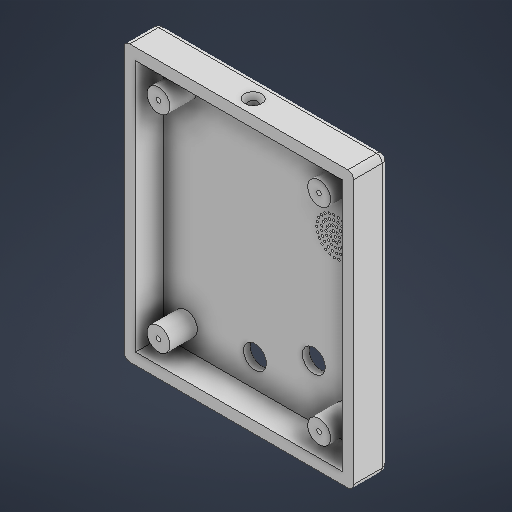
# Autodesk Inventor part: Top_Shell
Saved by Autodesk Inventor 2026.2 (Build 302298010, 298A)
## iProperties
Created: 2026-03-03
Part Number: Top_Shell
Material: Generic
Document SubType Name: Modeling
Designer: kjedr
Density: 1 g/cm^3
Appearance: Default
Author: kjedr
Autodesk Inventor part; units mm, degrees
ref_plane "YZ Plane" through (0, 0, 0) normal (1, 0, 0) x (0, 1, 0)
ref_plane "XZ Plane" through (0, 0, 0) normal (0, 1, 0) x (-1, 0, 0)
ref_plane "XY Plane" through (0, 0, 0) normal (0, 0, 1) x (1, 0, 0)
sketch "Sketch1" plane through (0, 0, 0) normal (0, 0, 1) x (1, 0, 0)
  line L0 (0, 0) -> (127, 0)
  line L1 (127, 0) -> (127, 152.4)
  line L2 (127, 152.4) -> (0, 152.4)
  line L3 (0, 152.4) -> (0, 0)
  dimension "d0" = 127
  dimension "d1" = 152.4
  constraints: 8 end point, 2 parallel, 1 horizontal, 1 perpendicular
  measures "d0" distance of L2.end L1.end
  measures "d1" distance of L1.end L0.end
extrude "Extrusion1" add sketch "Sketch1" along normal blind 19.05
sketch "Sketch2" plane through (0, 0, 19.05) normal (0, 0, 1) x (1, 0, 0)
  line L0 (6.35, 6.35) -> (120.65, 6.35)
  line L1 (120.65, 6.35) -> (120.65, 146.05)
  line L2 (120.65, 146.05) -> (6.35, 146.05)
  line L3 (6.35, 146.05) -> (6.35, 6.35)
  line L4 (0, 152.4) -> (0, 0) projected
  line L5 (0, 0) -> (127, 0) projected
  line L6 (127, 0) -> (127, 152.4) projected
  line L7 (127, 152.4) -> (0, 152.4) projected
  point P0 (127, 76.2)
  dimension "d4" = 6.35
  dimension "d5" = 6.35
  dimension "d6" = 6.35
  dimension "d7" = 6.35
  constraints: 8 end point, 2 parallel, 1 horizontal, 1 midpoint, 1 perpendicular
  measures "d4" distance between parallel lines of L4 L3
  measures "d5" distance between parallel lines of L5 L0
  measures "d6" distance from line of point (127, 76.2) L1
  measures "d7" distance between parallel lines of L7 L2
extrude "Extrusion2" cut sketch "Sketch2" against normal blind 15.24 contours L3 L2 L1 L0
sketch "Sketch3" plane through (0, 0, 3.81) normal (0, 0, 1) x (1, 0, 0)
  circle A0 centre (19.05, 133.35) radius 6.35
  circle A1 centre (107.95, 133.35) radius 6.35
  circle A2 centre (19.05, 19.05) radius 6.35
  circle A3 centre (107.95, 19.05) radius 6.35
  line L0 (6.35, 6.35) -> (6.35, 146.05) projected
  line L1 (6.35, 146.05) -> (120.65, 146.05) projected
  line L2 (120.65, 6.35) -> (6.35, 6.35) projected
  line L3 (120.65, 146.05) -> (120.65, 6.35) projected
  point P0 (0, 0)
  dimension "d10" = 12.7
  dimension "d11" = 12.7
  dimension "d12" = 12.7
  dimension "d13" = 12.7
  dimension "d14" = 12.7
  constraints: 4 centre point, 3 equal radius, 2 horizontal alignment, 2 vertical alignment
  measures "d10" distance from line of L0 A0.centre
  measures "d11" distance from line of L1 A0.centre
  measures "d12" distance from line of L2 A2.centre
  measures "d13" distance from line of L3 A1.centre
  measures "d14" diameter of A0
extrude "Extrusion3" add sketch "Sketch3" along normal up to surface (15.24 mm away) contours A0 | A1 | A2 | A3
fillet "Fillet1" radius 3.175 8 edges at (127, 152.4, 9.525) (0, 152.4, 9.525) (63.5, 152.4, 0) (127, 76.2, 0) (63.5, 0, 0) (0, 76.2, 0) (0, 0, 9.525) (127, 0, 9.525)
sketch "Sketch8" plane through (0, 0, 0) normal (0, 0, -1) x (-1, 0, 0)
  circle A0 centre (-101.6, 101.6) radius 12.7 construction
  circle A1 centre (-101.6, 101.6) radius 10.16 construction
  circle A2 centre (-101.6, 101.6) radius 7.62 construction
  circle A3 centre (-101.6, 101.6) radius 5.08 construction
  circle A4 centre (-101.6, 101.6) radius 2.54 construction
  line L0 (-127, 149.225) -> (-127, 3.175) projected
  line L1 (-123.825, 0) -> (-3.175, 0) projected
  point P0 (0, 0)
  point P1 (-100.7328, 103.9874)
  point P2 (-102.5144, 106.597)
  point P3 (-100.8008, 109.178)
  point P4 (-100.7838, 111.7272)
  point P5 (-103.328, 111.612)
  point P6 (-105.7636, 110.8677)
  point P7 (-107.9376, 109.5411)
  point P8 (-109.7133, 107.7155)
  point P9 (-110.9793, 105.5057)
  point P10 (-111.6559, 103.0504)
  point P11 (-111.7007, 100.5041)
  point P12 (-111.1108, 98.0266)
  point P13 (-109.9234, 95.7736)
  point P14 (-108.2129, 93.8867)
  point P15 (-106.0869, 92.4845)
  point P16 (-103.679, 91.655)
  point P17 (-101.1405, 91.4504)
  point P18 (-98.6308, 91.8835)
  point P19 (-96.3077, 92.9272)
  point P20 (-94.3171, 94.5158)
  point P21 (-92.7842, 96.5496)
  point P22 (-91.8051, 98.9006)
  point P23 (-91.4416, 101.4213)
  point P24 (-91.7163, 103.9532)
  point P25 (-92.612, 106.3373)
  point P26 (-94.0725, 108.4237)
  point P27 (-96.006, 110.0813)
  point P28 (-98.2909, 111.206)
  point P29 (-103.1817, 109.054)
  point P30 (-105.4077, 108.2004)
  point P31 (-107.261, 106.7008)
  point P32 (-108.5601, 104.7018)
  point P33 (-109.178, 102.3992)
  point P34 (-109.054, 100.0183)
  point P35 (-108.2004, 97.7923)
  point P36 (-106.7008, 95.939)
  point P37 (-104.7018, 94.6399)
  point P38 (-102.3992, 94.022)
  point P39 (-100.0183, 94.146)
  point P40 (-97.7923, 94.9996)
  point P41 (-95.939, 96.4992)
  point P42 (-94.6399, 98.4982)
  point P43 (-94.022, 100.8008)
  point P44 (-94.146, 103.1817)
  point P45 (-94.9996, 105.4077)
  point P46 (-96.4992, 107.261)
  point P47 (-98.4982, 108.5601)
  point P48 (-104.4678, 105.7931)
  point P49 (-105.9254, 104.2641)
  point P50 (-106.635, 102.2745)
  point P51 (-106.4741, 100.1682)
  point P52 (-105.4703, 98.3096)
  point P53 (-103.7974, 97.0198)
  point P54 (-101.7445, 96.5221)
  point P55 (-99.6666, 96.9023)
  point P56 (-97.923, 98.0948)
  point P57 (-96.8152, 99.8934)
  point P58 (-96.5348, 101.9871)
  point P59 (-97.1301, 104.0138)
  point P60 (-98.4984, 105.6232)
  point P61 (-100.4029, 106.5369)
  point P62 (-102.675, 103.9013)
  point P63 (-103.9874, 102.4672)
  point P64 (-103.9013, 100.525)
  point P65 (-102.4672, 99.2126)
  point P66 (-100.525, 99.2987)
  point P67 (-99.2126, 100.7328)
  point P68 (-99.2987, 102.675)
  dimension "d39" = 20.32
  dimension "d40" = 15.24
  dimension "d41" = 10.16
  dimension "d42" = 5.08
  dimension "d38" = 25.4
  dimension "d45" = 360
  dimension "d49" = 360
  dimension "d53" = 360
  dimension "d57" = 360
  dimension "d66" = 25.4
  dimension "d67" = 101.6
  constraints: 5 coincident, 1 centre point, 84 other
  measures "d38" diameter of A0
  measures "d66" distance from line of L0 A0.centre
  measures "d67" distance from line of L1 A0.centre
hole "Hole1" at (101.6, 101.6, 0) at (100.7328, 103.9874, 0) at (102.5144, 106.597, 0) at (100.8008, 109.178, 0) at (100.7838, 111.7272, 0) at (103.328, 111.612, 0) at (105.7636, 110.8677, 0) at (107.9376, 109.5411, 0) at (109.7133, 107.7155, 0) at (110.9793, 105.5057, 0) at (111.6559, 103.0504, 0) at (111.7007, 100.5041, 0) at (111.1108, 98.0266, 0) at (109.9234, 95.7736, 0) at (108.2129, 93.8867, 0) at (106.0869, 92.4845, 0) at (103.679, 91.655, 0) at (101.1405, 91.4504, 0) at (98.6308, 91.8835, 0) at (96.3077, 92.9272, 0) at (94.3171, 94.5158, 0) at (92.7842, 96.5496, 0) at (91.8051, 98.9006, 0) at (91.4416, 101.4213, 0) at (91.7163, 103.9532, 0) at (92.612, 106.3373, 0) at (94.0725, 108.4237, 0) at (96.006, 110.0813, 0) at (98.2909, 111.206, 0) at (103.1817, 109.054, 0) at (105.4077, 108.2004, 0) at (107.261, 106.7008, 0) at (108.5601, 104.7018, 0) at (109.178, 102.3992, 0) at (109.054, 100.0183, 0) at (108.2004, 97.7923, 0) at (106.7008, 95.939, 0) at (104.7018, 94.6399, 0) at (102.3992, 94.022, 0) at (100.0183, 94.146, 0) at (97.7923, 94.9996, 0) at (95.939, 96.4992, 0) at (94.6399, 98.4982, 0) at (94.022, 100.8008, 0) at (94.146, 103.1817, 0) at (94.9996, 105.4077, 0) at (96.4992, 107.261, 0) at (98.4982, 108.5601, 0) at (104.4678, 105.7931, 0) at (105.9254, 104.2641, 0) direction (0, 0, 1) diameter 1.27 end through all and at (106.635, 102.2745, 0) (106.4741, 100.1682, 0) (105.4703, 98.3096, 0) (103.7974, 97.0198, 0) (101.7445, 96.5221, 0) (99.6666, 96.9023, 0) (97.923, 98.0948, 0) (96.8152, 99.8934, 0) (96.5348, 101.9871, 0) (97.1301, 104.0138, 0) (98.4984, 105.6232, 0) (100.4029, 106.5369, 0) (102.675, 103.9013, 0) (103.9874, 102.4672, 0) (103.9013, 100.525, 0) (102.4672, 99.2126, 0) (100.525, 99.2987, 0) (99.2126, 100.7328, 0) (99.2987, 102.675, 0)
sketch "Sketch9" plane through (0, 0, 3.81) normal (0, 0, 1) x (1, 0, 0)
  line L0 (87.63, 115.57) -> (115.57, 115.57)
  line L1 (115.57, 115.57) -> (115.57, 87.63)
  line L2 (115.57, 87.63) -> (87.63, 87.63)
  line L3 (87.63, 87.63) -> (87.63, 115.57)
  circle A0 centre (101.6, 101.6) radius 0.635 projected
  line L4 (87.63, 115.57) -> (115.57, 87.63) construction
  line L5 (115.57, 115.57) -> (87.63, 87.63) construction
  point P0 (0, 0)
  dimension "d68" = 27.94
  dimension "d69" = 27.94
  constraints: 12 end point, 2 midpoint, 2 parallel, 1 horizontal, 1 perpendicular
  measures "d68" distance of L1.end L2.end
  measures "d69" distance of L0.end L1.end
sketch "Sketch10" plane through (3.175, 152.4, 19.05) normal (0, 1, 0) x (1, 0, 0)
  line L0 (0, 15.875) -> (120.65, 15.875) projected
  point P0 (-3.175, 19.05)
  point P1 (60.325, 7.9375)
  point P2 (60.325, 15.875)
  constraints: 1 midpoint, 1 vertical alignment
hole "Hole2" at (63.5, 152.4, 11.1125) direction (0, -1, 0) diameter 5.08 depth 6.35 tip angle 118 countersink diameter 9.525 countersink angle 82
sketch "Sketch11" plane through (19.05, 19.05, 19.05) normal (0, 0, 1) x (1, 0, 0)
  circle A0 centre (0, 114.3) radius 6.35 projected
  circle A1 centre (88.9, 114.3) radius 6.35 projected
  circle A2 centre (0, 0) radius 6.35 projected
  circle A3 centre (88.9, 0) radius 6.35 projected
  point P0 (-19.05, -19.05)
  constraints: 4 coincident
hole "Hole3" at (19.05, 19.05, 19.05) at (19.05, 133.35, 19.05) at (107.95, 133.35, 19.05) at (107.95, 19.05, 19.05) direction (0, 0, -1) diameter 2.54 depth 12.7 tip angle 118
sketch "Sketch12" plane through (0, 0, 0) normal (0, 0, -1) x (-1, 0, 0)
  point P0 (0, 0)
sketch "Sketch13" plane through (0, 0, 0) normal (0, 0, -1) x (-1, 0, 0)
  circle A0 centre (-24.7536, 119.7454) radius 3.175
  point P0 (0, 0)
  dimension "d87" = 6.35
  constraints: 1 centre point
  measures "d87" diameter of A0
sketch "Sketch14" plane through (0, 0, 0) normal (0, 0, -1) x (-1, 0, 0)
  line L0 (-98.769, 93.35) -> (-28.231, 93.35) construction
  line L1 (-28.231, 93.35) -> (-28.231, 9.35) construction
  line L2 (-28.231, 9.35) -> (-98.769, 9.35) construction
  line L3 (-98.769, 9.35) -> (-98.769, 93.35) construction
  circle A0 centre (-94.2972, 86.056) radius 1.6
  circle A1 centre (-32.6768, 86.056) radius 1.6
  circle A2 centre (-94.2972, 25.35) radius 1.6
  circle A3 centre (-32.6768, 25.35) radius 1.6
  line L4 (-123.825, 149.225) -> (-3.175, 149.225) projected
  line L5 (-120.65, 6.35) -> (-6.35, 6.35) projected
  point P0 (0, 0)
  point P1 (-63.5, 93.35)
  point P2 (-63.5, 128.3133)
  point P3 (-89.789, 36.35)
  point P4 (-57.231, 21.85)
  point P5 (-63.5, 9.35)
  point P6 (-63.5, 149.225)
  dimension "d88" = 70.538
  dimension "d89" = 84
  dimension "d90" = 3.2
  dimension "d91" = 60.706
  dimension "d92" = 61.6204
  dimension "d93" = 16
  dimension "d94" = 4.4458
  dimension "d96" = 27
  dimension "d97" = 8.98
  dimension "d98" = 12.5
  dimension "d99" = 29
  dimension "d101" = 3
  constraints: 8 end point, 4 centre point, 4 vertical alignment, 3 equal radius, 3 midpoint, 2 horizontal alignment, 2 parallel, 1 horizontal, 1 perpendicular
  measures "d88" distance of L1.end L2.end
  measures "d89" distance of L0.end L1.end
  measures "d90" diameter of A0
  measures "d91" distance of A2.centre A0.centre
  measures "d92" distance of A3.centre A2.centre
  measures "d93" distance from line of L2 A3.centre
  measures "d94" distance from line of L1 A3.centre
  measures "d96" distance from line of L2 point (-89.789, 36.35)
  measures "d97" distance from line of L3 point (-89.789, 36.35)
  measures "d98" distance from line of L2 point (-57.231, 21.85)
  measures "d99" distance from line of L1 point (-57.231, 21.85)
  measures "d101" distance between parallel lines of L5 L2
hole "Hole4" at (89.789, 36.35, 0) at (57.231, 21.85, 0) direction (0, 0, 1) diameter 12.7 end through all
body "Solid1"
